Autodesk Inventor part; units mm, degrees
(part 2 of 2)
extrude "Extrusion9" add sketch "Esquisse10" against normal blind 4.5 contours L101 A22 L104 | L101 L102 A22 | A22 L103 L104 | L102 L103 A22 | L109 A23 L112 | L109 L110 A23 | A23 L111 L112 | L110 L111 A23 | L135 A24 L138 | L135 L136 A24 | A24 L137 L138 | L136 L137 A24 | L143 A25 L146 | L143 L144 A25 | A25 L145 L146 | L144 L145 A25
extrude "Extrusion10" add sketch "Esquisse10" against normal blind 1.5 contours L97 A19 L100 | L97 L98 A19 | A19 L99 L100 | L98 L99 A19 | L105 A18 L108 | L105 L106 A18 | A18 L107 L108 | L106 L107 A18 | L139 A21 L142 | L139 L140 A21 | A21 L141 L142 | L140 L141 A21 | L147 A20 L150 | L147 L148 A20 | A20 L149 L150 | L148 L149 A20
sketch "Esquisse11" plane through (0, 0, 2.5) normal (0, 0, 1) x (1, 0, 0)
  arc A0 (-3.3524, 12) -> (-0.293, 24.5947) centre (-50, 30) ccw projected
  arc A1 (-0.293, 24.5947) -> (-1.5, 25) centre (-1.5, 23) ccw projected
  line L0 (-1.5, 25) -> (-18, 25) projected
  arc A2 (-18, 25) -> (-22, 21) centre (-18, 21) ccw projected
  line L1 (-22, 21) -> (-22, 16) projected
  arc A3 (-22, 16) -> (-18, 12) centre (-18, 16) ccw projected
  line L2 (-18, 12) -> (-3.3524, 12) projected
  circle A4 centre (-16.5, 17.5) radius 2.5 projected
  line L3 (-9, 15) -> (-9, 20) projected
  line L4 (-9, 20) -> (-4, 20) projected
  line L5 (-4, 20) -> (-4, 15) projected
  line L6 (-4, 15) -> (-9, 15) projected
  line L7 (-18, 35) -> (-1.5, 35) projected
  arc A5 (-1.5, 35) -> (-0.293, 35.4053) centre (-1.5, 37) ccw projected
  arc A6 (-0.293, 35.4053) -> (-3.3524, 48) centre (-50, 30) ccw projected
  line L8 (-3.3524, 48) -> (-18, 48) projected
  arc A7 (-18, 48) -> (-22, 44) centre (-18, 44) ccw projected
  line L9 (-22, 44) -> (-22, 39) projected
  arc A8 (-22, 39) -> (-18, 35) centre (-18, 39) ccw projected
  line L10 (-9, 40) -> (-9, 45) projected
  line L11 (-9, 45) -> (-4, 45) projected
  line L12 (-4, 45) -> (-4, 40) projected
  line L13 (-4, 40) -> (-9, 40) projected
  circle A9 centre (-16.5, 42.5) radius 2.5 projected
  circle A10 centre (-83.5, 42.5) radius 2.5 projected
  arc A11 (-78, 44) -> (-82, 48) centre (-82, 44) ccw projected
  line L14 (-82, 48) -> (-96.6476, 48) projected
  arc A12 (-96.6476, 48) -> (-99.707, 35.4053) centre (-50, 30) ccw projected
  arc A13 (-99.707, 35.4053) -> (-98.5, 35) centre (-98.5, 37) ccw projected
  line L15 (-98.5, 35) -> (-82, 35) projected
  arc A14 (-82, 35) -> (-78, 39) centre (-82, 39) ccw projected
  line L16 (-78, 39) -> (-78, 44) projected
  line L17 (-91, 45) -> (-91, 40) projected
  line L18 (-91, 40) -> (-96, 40) projected
  line L19 (-96, 40) -> (-96, 45) projected
  line L20 (-96, 45) -> (-91, 45) projected
  line L21 (-78, 16) -> (-78, 21) projected
  arc A15 (-78, 21) -> (-82, 25) centre (-82, 21) ccw projected
  line L22 (-82, 25) -> (-98.5, 25) projected
  arc A16 (-98.5, 25) -> (-99.707, 24.5947) centre (-98.5, 23) ccw projected
  arc A17 (-99.707, 24.5947) -> (-96.6476, 12) centre (-50, 30) ccw projected
  line L23 (-96.6476, 12) -> (-82, 12) projected
  arc A18 (-82, 12) -> (-78, 16) centre (-82, 16) ccw projected
  line L24 (-91, 20) -> (-91, 15) projected
  line L25 (-91, 15) -> (-96, 15) projected
  line L26 (-96, 15) -> (-96, 20) projected
  line L27 (-96, 20) -> (-91, 20) projected
  circle A19 centre (-83.5, 17.5) radius 2.5 projected
  circle A20 centre (-6.5, 17.5) radius 2.5
  circle A21 centre (-6.5, 42.5) radius 2.5
  circle A22 centre (-93.5, 42.5) radius 2.5
  circle A23 centre (-93.5, 17.5) radius 2.5
  point P0 (0, 0)
  constraints: 12 tangent, 4 centre point
extrude "Extrusion11" add sketch "Esquisse11" against normal blind 3 contours L3 A20 L6 | L3 L4 A20 | A20 L5 L6 | L4 L5 A20 | L10 A21 L13 | L10 L11 A21 | A21 L12 L13 | L11 L12 A21 | L17 A22 L20 | L17 L18 A22 | A22 L19 L20 | L18 L19 A22 | L24 A23 L27 | L24 L25 A23 | A23 L26 L27 | L25 L26 A23
